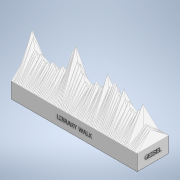
# Autodesk Inventor part: average_smplitude
Saved by Autodesk Inventor 2020 (Build 240168000, 168)
## iProperties
Created: 2019-09-30
Part Number: average_smplitude
Material: Generic
Document SubType Name: Modeling
Designer: Babynado
Density: 1 g/cm^3
Appearance: Default
Author: Babynado
Autodesk Inventor part; units mm, degrees
(part 1 of 3)
ref_plane "YZ Plane" through (0, 0, 0) normal (1, 0, 0) x (0, 1, 0)
ref_plane "XZ Plane" through (0, 0, 0) normal (0, 1, 0) x (-1, 0, 0)
ref_plane "XY Plane" through (0, 0, 0) normal (0, 0, 1) x (1, 0, 0)
sketch "Sketch1" plane through (0, 0, 0) normal (0, 1, 0) x (-1, 0, 0)
  line L0 (0, 0) -> (0, 50.8) projected
  line L1 (0, 50.8) -> (-203.2, 50.8) projected
  line L2 (-203.2, 50.8) -> (-203.2, 0) projected
  line L3 (-203.2, 0) -> (0, 0) projected
extrude "Extrusion1" add sketch "Sketch1" against normal blind 25.4
sketch "Sketch2" plane through (0, -25.4, 0) normal (0, -1, 0) x (1, 0, 0)
  line L0 (203.2, 0) -> (203.2, 50.8) projected
  line L1 (203.2, 50.8) -> (0, 50.8) projected
  line L2 (0, 50.8) -> (0, 0) projected
  line L3 (0, 0) -> (203.2, 0) projected
  line L4 (50.8, 29.464) -> (152.4, 29.464) construction
  line L5 (152.4, 29.464) -> (152.4, 21.336) construction
  line L6 (152.4, 21.336) -> (50.8, 21.336) construction
  line L7 (50.8, 21.336) -> (50.8, 29.464) construction
  spline S0 degree 2 poles (83.5812, 38.9215) (83.5812, 38.1212) (82.6031, 37.2517) (81.7781, 37.2517) knots 0 0 0 1 2 2 2
  spline S1 degree 2 poles (81.7781, 37.2517) (81.5805, 37.2517) (80.9235, 37.3209) (80.7012, 37.3703) knots 0 0 0 1 2 2 2
  line L8 (80.7012, 37.3703) -> (80.7012, 38.1508)
  line L9 (80.7012, 38.1508) -> (80.7457, 38.1508)
  spline S2 degree 2 poles (80.7457, 38.1508) (80.9136, 38.0915) (81.4126, 37.9532) (81.6694, 37.9532) knots 0 0 0 1 2 2 2
  spline S3 degree 2 poles (81.6694, 37.9532) (82.0449, 37.9532) (82.4944, 38.1261) (82.5982, 38.2842) knots 0 0 0 1 2 2 2
  spline S4 degree 2 poles (82.5982, 38.2842) (82.7118, 38.4472) (82.7711, 38.9215) (82.7711, 39.2327) knots 0 0 0 1 2 2 2
  line L10 (82.7711, 39.2327) -> (82.7711, 42.7846)
  line L11 (82.7711, 42.7846) -> (81.4817, 42.7846)
  line L12 (81.4817, 42.7846) -> (81.4817, 43.4317)
  line L13 (81.4817, 43.4317) -> (83.5812, 43.4317)
  line L14 (83.5812, 43.4317) -> (83.5812, 38.9215)
  line L15 (88.2743, 37.3357) -> (87.5036, 37.3357)
  line L16 (87.5036, 37.3357) -> (87.5036, 37.8396)
  spline S5 degree 2 poles (87.5036, 37.8396) (87.1479, 37.5284) (86.5107, 37.2073) (86.1155, 37.2073) knots 0 0 0 1 2 2 2
  spline S6 degree 2 poles (86.1155, 37.2073) (85.8191, 37.2073) (85.2905, 37.4049) (85.0978, 37.6173) knots 0 0 0 1 2 2 2
  spline S7 degree 2 poles (85.0978, 37.6173) (84.9002, 37.8297) (84.6829, 38.4769) (84.6829, 38.9412) knots 0 0 0 1 2 2 2
  line L17 (84.6829, 38.9412) -> (84.6829, 41.9102)
  line L18 (84.6829, 41.9102) -> (85.4535, 41.9102)
  line L19 (85.4535, 41.9102) -> (85.4535, 39.3019)
  spline S8 degree 2 poles (85.4535, 39.3019) (85.4535, 38.9363) (85.5078, 38.4571) (85.6017, 38.2793) knots 0 0 0 1 2 2 2
  spline S9 degree 2 poles (85.6017, 38.2793) (85.6956, 38.1014) (86.0167, 37.9384) (86.318, 37.9384) knots 0 0 0 1 2 2 2
  spline S10 degree 2 poles (86.318, 37.9384) (86.5996, 37.9384) (87.2369, 38.2595) (87.5036, 38.4917) knots 0 0 0 1 2 2 2
  line L20 (87.5036, 38.4917) -> (87.5036, 41.9102)
  line L21 (87.5036, 41.9102) -> (88.2743, 41.9102)
  line L22 (88.2743, 41.9102) -> (88.2743, 37.3357)
  spline S11 degree 2 poles (90.6257, 37.227) (90.1663, 37.227) (89.3709, 37.474) (89.1091, 37.6124) knots 0 0 0 1 2 2 2
  line L23 (89.1091, 37.6124) -> (89.1091, 38.4769)
  line L24 (89.1091, 38.4769) -> (89.1486, 38.4769)
  spline S12 degree 2 poles (89.1486, 38.4769) (89.2474, 38.3978) (89.5142, 38.2101) (89.7365, 38.1064) knots 0 0 0 1 2 2 2
  spline S13 degree 2 poles (89.7365, 38.1064) (89.9292, 38.0125) (90.4034, 37.8742) (90.6554, 37.8742) knots 0 0 0 1 2 2 2
  spline S14 degree 2 poles (90.6554, 37.8742) (90.8381, 37.8742) (91.258, 37.9582) (91.3568, 38.0273) knots 0 0 0 1 2 2 2
  spline S15 degree 2 poles (91.3568, 38.0273) (91.5001, 38.1212) (91.6285, 38.3336) (91.6285, 38.551) knots 0 0 0 1 2 2 2
  spline S16 degree 2 poles (91.6285, 38.551) (91.6285, 38.8227) (91.3321, 39.1043) (90.9518, 39.1981) knots 0 0 0 1 2 2 2
  spline S17 degree 2 poles (90.9518, 39.1981) (90.8036, 39.2327) (90.3293, 39.3315) (90.1268, 39.3858) knots 0 0 0 1 2 2 2
  spline S18 degree 2 poles (90.1268, 39.3858) (89.6031, 39.539) (89.1289, 40.1713) (89.1289, 40.6208) knots 0 0 0 1 2 2 2
  spline S19 degree 2 poles (89.1289, 40.6208) (89.1289, 41.2433) (90.0626, 42.0189) (90.8332, 42.0189) knots 0 0 0 1 2 2 2
  spline S20 degree 2 poles (90.8332, 42.0189) (91.2136, 42.0189) (91.9842, 41.8312) (92.246, 41.6879) knots 0 0 0 1 2 2 2
  line L25 (92.246, 41.6879) -> (92.246, 40.8629)
  line L26 (92.246, 40.8629) -> (92.2065, 40.8629)
  spline S21 degree 2 poles (92.2065, 40.8629) (91.9101, 41.1) (91.1889, 41.3717) (90.8184, 41.3717) knots 0 0 0 1 2 2 2
  spline S22 degree 2 poles (90.8184, 41.3717) (90.438, 41.3717) (89.9144, 41.0506) (89.9144, 40.7295) knots 0 0 0 1 2 2 2
  spline S23 degree 2 poles (89.9144, 40.7295) (89.9144, 40.4381) (90.2256, 40.1565) (90.5714, 40.0676) knots 0 0 0 1 2 2 2
  spline S24 degree 2 poles (90.5714, 40.0676) (90.7393, 40.0231) (91.1642, 39.9342) (91.3964, 39.8798) knots 0 0 0 1 2 2 2
  spline S25 degree 2 poles (91.3964, 39.8798) (91.9002, 39.7514) (92.414, 39.1635) (92.414, 38.6547) knots 0 0 0 1 2 2 2
  spline S26 degree 2 poles (92.414, 38.6547) (92.414, 38.3583) (92.1818, 37.8347) (91.9546, 37.642) knots 0 0 0 1 2 2 2
  spline S27 degree 2 poles (91.9546, 37.642) (91.7125, 37.4395) (91.095, 37.227) (90.6257, 37.227) knots 0 0 0 1 2 2 2
  spline S28 degree 2 poles (94.5135, 37.2468) (93.8861, 37.2468) (93.1797, 37.9631) (93.1797, 38.7387) knots 0 0 0 1 2 2 2
  line L27 (93.1797, 38.7387) -> (93.1797, 41.2729)
  line L28 (93.1797, 41.2729) -> (92.661, 41.2729)
  line L29 (92.661, 41.2729) -> (92.661, 41.9102)
  line L30 (92.661, 41.9102) -> (93.1797, 41.9102)
  line L31 (93.1797, 41.9102) -> (93.1797, 43.2242)
  line L32 (93.1797, 43.2242) -> (93.9504, 43.2242)
  line L33 (93.9504, 43.2242) -> (93.9504, 41.9102)
  line L34 (93.9504, 41.9102) -> (95.3681, 41.9102)
  line L35 (95.3681, 41.9102) -> (95.3681, 41.2729)
  line L36 (95.3681, 41.2729) -> (93.9504, 41.2729)
  line L37 (93.9504, 41.2729) -> (93.9504, 39.0944)
  spline S29 degree 2 poles (93.9504, 39.0944) (93.9504, 38.7486) (93.9751, 38.3682) (94.059, 38.2052) knots 0 0 0 1 2 2 2
  spline S30 degree 2 poles (94.059, 38.2052) (94.1282, 38.0619) (94.4394, 37.9186) (94.7062, 37.9186) knots 0 0 0 1 2 2 2
  spline S31 degree 2 poles (94.7062, 37.9186) (94.8939, 37.9186) (95.2446, 38.0323) (95.3237, 38.0668) knots 0 0 0 1 2 2 2
  line L38 (95.3237, 38.0668) -> (95.3681, 38.0668)
  line L39 (95.3681, 38.0668) -> (95.3681, 37.3752)
  spline S32 degree 2 poles (95.3681, 37.3752) (95.1508, 37.316) (94.7062, 37.2468) (94.5135, 37.2468) knots 0 0 0 1 2 2 2
  line L40 (96.7217, 37.3357) -> (95.9511, 37.3357)
  line L41 (95.9511, 37.3357) -> (95.9511, 41.9102)
  line L42 (95.9511, 41.9102) -> (96.7217, 41.9102)
  line L43 (96.7217, 41.9102) -> (96.7217, 37.3357)
  line L44 (96.7761, 42.671) -> (95.9017, 42.671)
  line L45 (95.9017, 42.671) -> (95.9017, 43.4712)
  line L46 (95.9017, 43.4712) -> (96.7761, 43.4712)
  line L47 (96.7761, 43.4712) -> (96.7761, 42.671)
  line L48 (101.4444, 37.3357) -> (100.6737, 37.3357)
  line L49 (100.6737, 37.3357) -> (100.6737, 39.9441)
  spline S33 degree 2 poles (100.6737, 39.9441) (100.6737, 40.2602) (100.6145, 40.8036) (100.5255, 40.9666) knots 0 0 0 1 2 2 2
  spline S34 degree 2 poles (100.5255, 40.9666) (100.4317, 41.1395) (100.0958, 41.3075) (99.8092, 41.3075) knots 0 0 0 1 2 2 2
  spline S35 degree 2 poles (99.8092, 41.3075) (99.5227, 41.3075) (98.9151, 41.0012) (98.6236, 40.7542) knots 0 0 0 1 2 2 2
  line L50 (98.6236, 40.7542) -> (98.6236, 37.3357)
  line L51 (98.6236, 37.3357) -> (97.853, 37.3357)
  line L52 (97.853, 37.3357) -> (97.853, 41.9102)
  line L53 (97.853, 41.9102) -> (98.6236, 41.9102)
  line L54 (98.6236, 41.9102) -> (98.6236, 41.4014)
  spline S36 degree 2 poles (98.6236, 41.4014) (98.9694, 41.7126) (99.6363, 42.0386) (100.0118, 42.0386) knots 0 0 0 1 2 2 2
  spline S37 degree 2 poles (100.0118, 42.0386) (100.6836, 42.0386) (101.4444, 41.1494) (101.4444, 40.3047) knots 0 0 0 1 2 2 2
  line L55 (101.4444, 40.3047) -> (101.4444, 37.3357)
  line L56 (104.5467, 37.3357) -> (106.6018, 43.4317)
  line L57 (106.6018, 43.4317) -> (107.5997, 43.4317)
  line L58 (107.5997, 43.4317) -> (109.6547, 37.3357)
  line L59 (109.6547, 37.3357) -> (108.8001, 37.3357)
  line L60 (108.8001, 37.3357) -> (108.2468, 39.04)
  line L61 (108.2468, 39.04) -> (105.9201, 39.04)
  line L62 (105.9201, 39.04) -> (105.3668, 37.3357)
  line L63 (105.3668, 37.3357) -> (104.5467, 37.3357)
  line L64 (108.0245, 39.7316) -> (107.081, 42.6018)
  line L65 (107.081, 42.6018) -> (106.1424, 39.7316)
  line L66 (106.1424, 39.7316) -> (108.0245, 39.7316)
  line L67 (110.9589, 37.3357) -> (110.1882, 37.3357)
  line L68 (110.1882, 37.3357) -> (110.1882, 43.7034)
  line L69 (110.1882, 43.7034) -> (110.9589, 43.7034)
  line L70 (110.9589, 43.7034) -> (110.9589, 37.3357)
  line L71 (112.8756, 37.3357) -> (112.105, 37.3357)
  line L72 (112.105, 37.3357) -> (112.105, 43.7034)
  line L73 (112.105, 43.7034) -> (112.8756, 43.7034)
  line L74 (112.8756, 43.7034) -> (112.8756, 37.3357)
  spline S38 degree 2 poles (115.9928, 37.232) (114.8961, 37.232) (113.6907, 38.4621) (113.6907, 39.5983) knots 0 0 0 1 2 2 2
  spline S39 degree 2 poles (113.6907, 39.5983) (113.6907, 40.7147) (114.8615, 42.0386) (115.8051, 42.0386) knots 0 0 0 1 2 2 2
  spline S40 degree 2 poles (115.8051, 42.0386) (116.2299, 42.0386) (116.8869, 41.7916) (117.129, 41.5298) knots 0 0 0 1 2 2 2
  spline S41 degree 2 poles (117.129, 41.5298) (117.376, 41.268) (117.6378, 40.5122) (117.6378, 39.9638) knots 0 0 0 1 2 2 2
  line L75 (117.6378, 39.9638) -> (117.6378, 39.5439)
  line L76 (117.6378, 39.5439) -> (114.4713, 39.5439)
  spline S42 degree 2 poles (114.4713, 39.5439) (114.4713, 38.7486) (115.2715, 37.9038) (115.9829, 37.9038) knots 0 0 0 1 2 2 2
  spline S43 degree 2 poles (115.9829, 37.9038) (116.2348, 37.9038) (116.7239, 38.0174) (116.9215, 38.1064) knots 0 0 0 1 2 2 2
  spline S44 degree 2 poles (116.9215, 38.1064) (117.129, 38.2052) (117.4155, 38.3781) (117.5094, 38.4571) knots 0 0 0 1 2 2 2
  line L77 (117.5094, 38.4571) -> (117.5538, 38.4571)
  line L78 (117.5538, 38.4571) -> (117.5538, 37.6173)
  spline S45 degree 2 poles (117.5538, 37.6173) (117.4205, 37.563) (117.0154, 37.4049) (116.8573, 37.3604) knots 0 0 0 1 2 2 2
  spline S46 degree 2 poles (116.8573, 37.3604) (116.635, 37.2962) (116.2694, 37.232) (115.9928, 37.232) knots 0 0 0 1 2 2 2
  spline S47 degree 2 poles (116.8869, 40.1318) (116.877, 40.443) (116.7486, 40.8975) (116.6251, 41.0506) knots 0 0 0 1 2 2 2
  spline S48 degree 2 poles (116.6251, 41.0506) (116.4917, 41.2235) (116.0718, 41.4063) (115.7606, 41.4063) knots 0 0 0 1 2 2 2
  spline S49 degree 2 poles (115.7606, 41.4063) (115.4543, 41.4063) (115.0245, 41.2235) (114.8467, 41.0457) knots 0 0 0 1 2 2 2
  spline S50 degree 2 poles (114.8467, 41.0457) (114.6738, 40.8629) (114.496, 40.4232) (114.4713, 40.1318) knots 0 0 0 1 2 2 2
  line L79 (114.4713, 40.1318) -> (116.8869, 40.1318)
  line L80 (122.0097, 37.3357) -> (121.2391, 37.3357)
  line L81 (121.2391, 37.3357) -> (121.2391, 39.9441)
  spline S51 degree 2 poles (121.2391, 39.9441) (121.2391, 40.2602) (121.1798, 40.8036) (121.0909, 40.9666) knots 0 0 0 1 2 2 2
  spline S52 degree 2 poles (121.0909, 40.9666) (120.997, 41.1395) (120.6611, 41.3075) (120.3746, 41.3075) knots 0 0 0 1 2 2 2
  spline S53 degree 2 poles (120.3746, 41.3075) (120.0881, 41.3075) (119.4804, 41.0012) (119.189, 40.7542) knots 0 0 0 1 2 2 2
  line L82 (119.189, 40.7542) -> (119.189, 37.3357)
  line L83 (119.189, 37.3357) -> (118.4183, 37.3357)
  line L84 (118.4183, 37.3357) -> (118.4183, 41.9102)
  line L85 (118.4183, 41.9102) -> (119.189, 41.9102)
  line L86 (119.189, 41.9102) -> (119.189, 41.4014)
  spline S54 degree 2 poles (119.189, 41.4014) (119.5348, 41.7126) (120.2017, 42.0386) (120.5771, 42.0386) knots 0 0 0 1 2 2 2
  spline S55 degree 2 poles (120.5771, 42.0386) (121.249, 42.0386) (122.0097, 41.1494) (122.0097, 40.3047) knots 0 0 0 1 2 2 2
  line L87 (122.0097, 40.3047) -> (122.0097, 37.3357)
  line L88 (80.7481, 27.2988) -> (82.8032, 33.3948)
  line L89 (82.8032, 33.3948) -> (83.8011, 33.3948)
  line L90 (83.8011, 33.3948) -> (85.8561, 27.2988)
  line L91 (85.8561, 27.2988) -> (85.0015, 27.2988)
  line L92 (85.0015, 27.2988) -> (84.4482, 29.0031)
  line L93 (84.4482, 29.0031) -> (82.1215, 29.0031)
  line L94 (82.1215, 29.0031) -> (81.5682, 27.2988)
  line L95 (81.5682, 27.2988) -> (80.7481, 27.2988)
  line L96 (84.2259, 29.6947) -> (83.2824, 32.5649)
  line L97 (83.2824, 32.5649) -> (82.3438, 29.6947)
  line L98 (82.3438, 29.6947) -> (84.2259, 29.6947)
  line L99 (89.7143, 27.2988) -> (86.7404, 27.2988)
  line L100 (86.7404, 27.2988) -> (86.7404, 27.9213)
  line L101 (86.7404, 27.9213) -> (87.8469, 27.9213)
  line L102 (87.8469, 27.9213) -> (87.8469, 32.0067)
  line L103 (87.8469, 32.0067) -> (86.7404, 32.0067)
  line L104 (86.7404, 32.0067) -> (86.7404, 32.5649)
  spline S56 degree 2 poles (86.7404, 32.5649) (87.3678, 32.5649) (87.9606, 32.9206) (88.0001, 33.4146) knots 0 0 0 1 2 2 2
  line L105 (88.0001, 33.4146) -> (88.6324, 33.4146)
  line L106 (88.6324, 33.4146) -> (88.6324, 27.9213)
  line L107 (88.6324, 27.9213) -> (89.7143, 27.9213)
  line L108 (89.7143, 27.9213) -> (89.7143, 27.2988)
  line L109 (94.7581, 29.3934) -> (94.0319, 29.3934)
  line L110 (94.0319, 29.3934) -> (94.0319, 27.2988)
  line L111 (94.0319, 27.2988) -> (93.2464, 27.2988)
  line L112 (93.2464, 27.2988) -> (93.2464, 29.3934)
  line L113 (93.2464, 29.3934) -> (90.5541, 29.3934)
  line L114 (90.5541, 29.3934) -> (90.5541, 30.253)
  line L115 (90.5541, 30.253) -> (93.281, 33.3948)
  line L116 (93.281, 33.3948) -> (94.0319, 33.3948)
  line L117 (94.0319, 33.3948) -> (94.0319, 30.0504)
  line L118 (94.0319, 30.0504) -> (94.7581, 30.0504)
  line L119 (94.7581, 30.0504) -> (94.7581, 29.3934)
  line L120 (93.2464, 30.0504) -> (93.2464, 32.4315)
  line L121 (93.2464, 32.4315) -> (91.1963, 30.0504)
  line L122 (91.1963, 30.0504) -> (93.2464, 30.0504)
  spline S57 degree 2 poles (99.1053, 29.2353) (99.1053, 28.7957) (98.8237, 28.0448) (98.5668, 27.7681) knots 0 0 0 1 2 2 2
  spline S58 degree 2 poles (98.5668, 27.7681) (98.3099, 27.4915) (97.5442, 27.1704) (97.07, 27.1704) knots 0 0 0 1 2 2 2
  spline S59 degree 2 poles (97.07, 27.1704) (96.6353, 27.1704) (95.7856, 27.363) (95.4744, 27.5162) knots 0 0 0 1 2 2 2
  line L123 (95.4744, 27.5162) -> (95.4744, 28.3807)
  line L124 (95.4744, 28.3807) -> (95.5336, 28.3807)
  spline S60 degree 2 poles (95.5336, 28.3807) (95.6275, 28.3115) (95.9782, 28.1337) (96.1907, 28.0546) knots 0 0 0 1 2 2 2
  spline S61 degree 2 poles (96.1907, 28.0546) (96.4327, 27.9707) (96.8329, 27.8768) (97.0848, 27.8768) knots 0 0 0 1 2 2 2
  spline S62 degree 2 poles (97.0848, 27.8768) (97.3318, 27.8768) (97.7962, 28.0546) (97.9641, 28.2473) knots 0 0 0 1 2 2 2
  spline S63 degree 2 poles (97.9641, 28.2473) (98.1173, 28.4301) (98.2754, 28.9142) (98.2754, 29.2403) knots 0 0 0 1 2 2 2
  spline S64 degree 2 poles (98.2754, 29.2403) (98.2754, 29.5663) (98.0975, 29.9813) (97.9296, 30.1196) knots 0 0 0 1 2 2 2
  spline S65 degree 2 poles (97.9296, 30.1196) (97.7567, 30.2727) (97.2429, 30.4012) (96.9317, 30.4012) knots 0 0 0 1 2 2 2
  spline S66 degree 2 poles (96.9317, 30.4012) (96.5957, 30.4012) (95.9288, 30.2974) (95.7263, 30.253) knots 0 0 0 1 2 2 2
  line L125 (95.7263, 30.253) -> (95.7263, 33.3948)
  line L126 (95.7263, 33.3948) -> (99.0707, 33.3948)
  line L127 (99.0707, 33.3948) -> (99.0707, 32.6785)
  line L128 (99.0707, 32.6785) -> (96.5118, 32.6785)
  line L129 (96.5118, 32.6785) -> (96.5118, 31.0532)
  spline S67 degree 2 poles (96.5118, 31.0532) (96.66, 31.073) (96.9465, 31.0878) (97.065, 31.0878) knots 0 0 0 1 2 2 2
  spline S68 degree 2 poles (97.065, 31.0878) (97.5344, 31.0878) (98.1815, 30.9347) (98.4779, 30.7074) knots 0 0 0 1 2 2 2
  spline S69 degree 2 poles (98.4779, 30.7074) (98.7792, 30.4802) (99.1053, 29.7886) (99.1053, 29.2353) knots 0 0 0 1 2 2 2
  spline S70 degree 2 poles (103.8378, 29.2748) (103.8378, 28.8055) (103.5266, 28.0102) (103.2648, 27.7434) knots 0 0 0 1 2 2 2
  spline S71 degree 2 poles (103.2648, 27.7434) (102.9931, 27.4618) (102.3114, 27.1704) (101.9013, 27.1704) knots 0 0 0 1 2 2 2
  spline S72 degree 2 poles (101.9013, 27.1704) (101.4913, 27.1704) (100.8145, 27.447) (100.5577, 27.7237) knots 0 0 0 1 2 2 2
  spline S73 degree 2 poles (100.5577, 27.7237) (100.2415, 28.0546) (99.8858, 29.1662) (99.8858, 29.9763) knots 0 0 0 1 2 2 2
  spline S74 degree 2 poles (99.8858, 29.9763) (99.8858, 30.7717) (100.2118, 32.0511) (100.5527, 32.5254) knots 0 0 0 1 2 2 2
  spline S75 degree 2 poles (100.5527, 32.5254) (100.8837, 32.9897) (101.931, 33.5084) (102.6176, 33.5084) knots 0 0 0 1 2 2 2
  spline S76 degree 2 poles (102.6176, 33.5084) (102.8202, 33.5084) (103.1759, 33.4689) (103.3093, 33.4245) knots 0 0 0 1 2 2 2
  line L130 (103.3093, 33.4245) -> (103.3093, 32.639)
  line L131 (103.3093, 32.639) -> (103.2747, 32.639)
  spline S77 degree 2 poles (103.2747, 32.639) (103.161, 32.6983) (102.7461, 32.802) (102.509, 32.802) knots 0 0 0 1 2 2 2
  spline S78 degree 2 poles (102.509, 32.802) (101.7482, 32.802) (100.8145, 31.7745) (100.7256, 30.7667) knots 0 0 0 1 2 2 2
  spline S79 degree 2 poles (100.7256, 30.7667) (101.0171, 30.9693) (101.6296, 31.1916) (101.9952, 31.1916) knots 0 0 0 1 2 2 2
  spline S80 degree 2 poles (101.9952, 31.1916) (102.3509, 31.1916) (102.8844, 31.0483) (103.1759, 30.8309) knots 0 0 0 1 2 2 2
  spline S81 degree 2 poles (103.1759, 30.8309) (103.5118, 30.579) (103.8378, 29.7985) (103.8378, 29.2748) knots 0 0 0 1 2 2 2
  spline S82 degree 2 poles (103.0079, 29.2403) (103.0079, 29.6157) (102.8103, 30.1245) (102.5929, 30.3024) knots 0 0 0 1 2 2 2
  spline S83 degree 2 poles (102.5929, 30.3024) (102.4299, 30.4308) (102.0248, 30.5148) (101.8124, 30.5148) knots 0 0 0 1 2 2 2
  spline S84 degree 2 poles (101.8124, 30.5148) (101.5259, 30.5148) (100.9874, 30.3419) (100.7256, 30.1789) knots 0 0 0 1 2 2 2
  spline S85 degree 2 poles (100.7256, 30.1789) (100.7207, 30.0899) (100.7108, 29.922) (100.7108, 29.7935) knots 0 0 0 1 2 2 2
  spline S86 degree 2 poles (100.7108, 29.7935) (100.7108, 29.1612) (100.9578, 28.3856) (101.1455, 28.1831) knots 0 0 0 1 2 2 2
  spline S87 degree 2 poles (101.1455, 28.1831) (101.3184, 27.9904) (101.6939, 27.8373) (101.9063, 27.8373) knots 0 0 0 1 2 2 2
  spline S88 degree 2 poles (101.9063, 27.8373) (102.4003, 27.8373) (103.0079, 28.5388) (103.0079, 29.2403) knots 0 0 0 1 2 2 2
  spline S89 degree 2 poles (108.4123, 29.2748) (108.4123, 28.8055) (108.1011, 28.0102) (107.8393, 27.7434) knots 0 0 0 1 2 2 2
  spline S90 degree 2 poles (107.8393, 27.7434) (107.5676, 27.4618) (106.8858, 27.1704) (106.4758, 27.1704) knots 0 0 0 1 2 2 2
  spline S91 degree 2 poles (106.4758, 27.1704) (106.0658, 27.1704) (105.389, 27.447) (105.1321, 27.7237) knots 0 0 0 1 2 2 2
  spline S92 degree 2 poles (105.1321, 27.7237) (104.816, 28.0546) (104.4603, 29.1662) (104.4603, 29.9763) knots 0 0 0 1 2 2 2
  spline S93 degree 2 poles (104.4603, 29.9763) (104.4603, 30.7717) (104.7863, 32.0511) (105.1272, 32.5254) knots 0 0 0 1 2 2 2
  spline S94 degree 2 poles (105.1272, 32.5254) (105.4582, 32.9897) (106.5055, 33.5084) (107.1921, 33.5084) knots 0 0 0 1 2 2 2
  spline S95 degree 2 poles (107.1921, 33.5084) (107.3947, 33.5084) (107.7503, 33.4689) (107.8837, 33.4245) knots 0 0 0 1 2 2 2
  line L132 (107.8837, 33.4245) -> (107.8837, 32.639)
  line L133 (107.8837, 32.639) -> (107.8491, 32.639)
  spline S96 degree 2 poles (107.8491, 32.639) (107.7355, 32.6983) (107.3206, 32.802) (107.0834, 32.802) knots 0 0 0 1 2 2 2
  spline S97 degree 2 poles (107.0834, 32.802) (106.3227, 32.802) (105.389, 31.7745) (105.3001, 30.7667) knots 0 0 0 1 2 2 2
  spline S98 degree 2 poles (105.3001, 30.7667) (105.5915, 30.9693) (106.2041, 31.1916) (106.5697, 31.1916) knots 0 0 0 1 2 2 2
  spline S99 degree 2 poles (106.5697, 31.1916) (106.9254, 31.1916) (107.4589, 31.0483) (107.7503, 30.8309) knots 0 0 0 1 2 2 2
  spline S100 degree 2 poles (107.7503, 30.8309) (108.0863, 30.579) (108.4123, 29.7985) (108.4123, 29.2748) knots 0 0 0 1 2 2 2
  spline S101 degree 2 poles (107.5824, 29.2403) (107.5824, 29.6157) (107.3848, 30.1245) (107.1674, 30.3024) knots 0 0 0 1 2 2 2
  spline S102 degree 2 poles (107.1674, 30.3024) (107.0044, 30.4308) (106.5993, 30.5148) (106.3869, 30.5148) knots 0 0 0 1 2 2 2
  spline S103 degree 2 poles (106.3869, 30.5148) (106.1004, 30.5148) (105.5619, 30.3419) (105.3001, 30.1789) knots 0 0 0 1 2 2 2
  spline S104 degree 2 poles (105.3001, 30.1789) (105.2951, 30.0899) (105.2853, 29.922) (105.2853, 29.7935) knots 0 0 0 1 2 2 2
  spline S105 degree 2 poles (105.2853, 29.7935) (105.2853, 29.1612) (105.5323, 28.3856) (105.72, 28.1831) knots 0 0 0 1 2 2 2
  spline S106 degree 2 poles (105.72, 28.1831) (105.8929, 27.9904) (106.2683, 27.8373) (106.4808, 27.8373) knots 0 0 0 1 2 2 2
  spline S107 degree 2 poles (106.4808, 27.8373) (106.9748, 27.8373) (107.5824, 28.5388) (107.5824, 29.2403) knots 0 0 0 1 2 2 2
  spline S108 degree 2 poles (112.9275, 30.3468) (112.9275, 28.7067) (111.9741, 27.1704) (110.9811, 27.1704) knots 0 0 0 1 2 2 2
  spline S109 degree 2 poles (110.9811, 27.1704) (109.9734, 27.1704) (109.0298, 28.7364) (109.0298, 30.3419) knots 0 0 0 1 2 2 2
  spline S110 degree 2 poles (109.0298, 30.3419) (109.0298, 31.9919) (109.9832, 33.5183) (110.9811, 33.5183) knots 0 0 0 1 2 2 2
  spline S111 degree 2 poles (110.9811, 33.5183) (111.9839, 33.5183) (112.9275, 31.9375) (112.9275, 30.3468) knots 0 0 0 1 2 2 2
  spline S112 degree 2 poles (111.8802, 28.4894) (111.9988, 28.7907) (112.0976, 29.7194) (112.0976, 30.3468) knots 0 0 0 1 2 2 2
  spline S113 degree 2 poles (112.0976, 30.3468) (112.0976, 30.9742) (111.9988, 31.898) (111.8753, 32.2092) knots 0 0 0 1 2 2 2
  spline S114 degree 2 poles (111.8753, 32.2092) (111.7518, 32.5204) (111.322, 32.8415) (110.9811, 32.8415) knots 0 0 0 1 2 2 2
  spline S115 degree 2 poles (110.9811, 32.8415) (110.6403, 32.8415) (110.2006, 32.5204) (110.0722, 32.1993) knots 0 0 0 1 2 2 2
  spline S116 degree 2 poles (110.0722, 32.1993) (109.9487, 31.8881) (109.8597, 30.9396) (109.8597, 30.3419) knots 0 0 0 1 2 2 2
  spline S117 degree 2 poles (109.8597, 30.3419) (109.8597, 29.6997) (109.9388, 28.8401) (110.0672, 28.5042) knots 0 0 0 1 2 2 2
  spline S118 degree 2 poles (110.0672, 28.5042) (110.1858, 28.188) (110.6254, 27.8472) (110.9811, 27.8472) knots 0 0 0 1 2 2 2
  spline S119 degree 2 poles (110.9811, 27.8472) (111.317, 27.8472) (111.7567, 28.1683) (111.8802, 28.4894) knots 0 0 0 1 2 2 2
  line L134 (117.5365, 32.4809) -> (114.8986, 27.2988)
  line L135 (114.8986, 27.2988) -> (114.0291, 27.2988)
  line L136 (114.0291, 27.2988) -> (116.8153, 32.6785)
  line L137 (116.8153, 32.6785) -> (113.6685, 32.6785)
  line L138 (113.6685, 32.6785) -> (113.6685, 33.3948)
  line L139 (113.6685, 33.3948) -> (117.5365, 33.3948)
  line L140 (117.5365, 33.3948) -> (117.5365, 32.4809)
  line L141 (121.7356, 27.2988) -> (118.7617, 27.2988)
  line L142 (118.7617, 27.2988) -> (118.7617, 27.9213)
  line L143 (118.7617, 27.9213) -> (119.8682, 27.9213)
  line L144 (119.8682, 27.9213) -> (119.8682, 32.0067)
  line L145 (119.8682, 32.0067) -> (118.7617, 32.0067)
  line L146 (118.7617, 32.0067) -> (118.7617, 32.5649)
  spline S120 degree 2 poles (118.7617, 32.5649) (119.3891, 32.5649) (119.9819, 32.9206) (120.0214, 33.4146) knots 0 0 0 1 2 2 2
  line L147 (120.0214, 33.4146) -> (120.6537, 33.4146)
  line L148 (120.6537, 33.4146) -> (120.6537, 27.9213)
  line L149 (120.6537, 27.9213) -> (121.7356, 27.9213)
  line L150 (121.7356, 27.9213) -> (121.7356, 27.2988)
  spline S121 degree 2 poles (70.8483, 17.1335) (70.8483, 16.353) (70.0085, 15.5329) (69.2724, 15.5329) knots 0 0 0 1 2 2 2
  spline S122 degree 2 poles (69.2724, 15.5329) (69.144, 15.5329) (68.8278, 15.5576) (68.6747, 15.5823) knots 0 0 0 1 2 2 2
  line L151 (68.6747, 15.5823) -> (68.6747, 16.2739)
  line L152 (68.6747, 16.2739) -> (68.7191, 16.2739)
  spline S123 degree 2 poles (68.7191, 16.2739) (68.8081, 16.2542) (69.0254, 16.2146) (69.1242, 16.2146) knots 0 0 0 1 2 2 2
  spline S124 degree 2 poles (69.1242, 16.2146) (69.4305, 16.2146) (69.8307, 16.3678) (69.9245, 16.5308) knots 0 0 0 1 2 2 2
  spline S125 degree 2 poles (69.9245, 16.5308) (70.0184, 16.679) (70.0777, 17.1285) (70.0777, 17.4496) knots 0 0 0 1 2 2 2
  line L153 (70.0777, 17.4496) -> (70.0777, 21.1991)
  line L154 (70.0777, 21.1991) -> (69.2527, 21.1991)
  line L155 (69.2527, 21.1991) -> (69.2527, 21.8364)
  line L156 (69.2527, 21.8364) -> (70.8483, 21.8364)
  line L157 (70.8483, 21.8364) -> (70.8483, 17.1335)
  line L158 (70.8532, 22.5972) -> (69.9789, 22.5972)
  line L159 (69.9789, 22.5972) -> (69.9789, 23.3974)
  line L160 (69.9789, 23.3974) -> (70.8532, 23.3974)
  line L161 (70.8532, 23.3974) -> (70.8532, 22.5972)
  spline S126 degree 2 poles (75.7982, 19.6233) (75.7982, 18.5019) (74.7114, 17.1335) (73.8914, 17.1335) knots 0 0 0 1 2 2 2
  spline S127 degree 2 poles (73.8914, 17.1335) (73.5209, 17.1335) (72.9923, 17.3163) (72.7354, 17.4743) knots 0 0 0 1 2 2 2
  line L162 (72.7354, 17.4743) -> (72.686, 17.2619)
  line L163 (72.686, 17.2619) -> (71.9647, 17.2619)
  line L164 (71.9647, 17.2619) -> (71.9647, 23.6296)
  line L165 (71.9647, 23.6296) -> (72.7354, 23.6296)
  line L166 (72.7354, 23.6296) -> (72.7354, 21.3572)
  spline S128 degree 2 poles (72.7354, 21.3572) (73.0269, 21.619) (73.7036, 21.9648) (74.1334, 21.9648) knots 0 0 0 1 2 2 2
  spline S129 degree 2 poles (74.1334, 21.9648) (74.909, 21.9648) (75.7982, 20.7249) (75.7982, 19.6233) knots 0 0 0 1 2 2 2
  spline S130 degree 2 poles (75.0029, 19.564) (75.0029, 20.384) (74.5039, 21.2337) (73.9506, 21.2337) knots 0 0 0 1 2 2 2
  spline S131 degree 2 poles (73.9506, 21.2337) (73.6394, 21.2337) (72.9972, 20.9373) (72.7354, 20.7101) knots 0 0 0 1 2 2 2
  line L167 (72.7354, 20.7101) -> (72.7354, 18.0869)
  spline S132 degree 2 poles (72.7354, 18.0869) (73.0269, 17.9436) (73.4764, 17.8251) (73.7432, 17.8251) knots 0 0 0 1 2 2 2
  spline S133 degree 2 poles (73.7432, 17.8251) (74.331, 17.8251) (75.0029, 18.6599) (75.0029, 19.564) knots 0 0 0 1 2 2 2
  spline S134 degree 2 poles (79.1476, 17.746) (79.0537, 17.6769) (78.7375, 17.4299) (78.5893, 17.3558) knots 0 0 0 1 2 2 2
  spline S135 degree 2 poles (78.5893, 17.3558) (78.3868, 17.2471) (78.0064, 17.1335) (77.6606, 17.1335) knots 0 0 0 1 2 2 2
  spline S136 degree 2 poles (77.6606, 17.1335) (77.379, 17.1335) (76.8702, 17.3459) (76.6775, 17.5386) knots 0 0 0 1 2 2 2
  spline S137 degree 2 poles (76.6775, 17.5386) (76.4948, 17.7263) (76.2725, 18.2796) (76.2725, 18.5858) knots 0 0 0 1 2 2 2
  spline S138 degree 2 poles (76.2725, 18.5858) (76.2725, 19.0601) (76.6726, 19.7319) (77.1073, 19.9246) knots 0 0 0 1 2 2 2
  spline S139 degree 2 poles (77.1073, 19.9246) (77.4926, 20.1024) (78.5399, 20.2358) (79.1476, 20.2704) knots 0 0 0 1 2 2 2
  line L168 (79.1476, 20.2704) -> (79.1476, 20.4186)
  spline S140 degree 2 poles (79.1476, 20.4186) (79.1476, 20.6854) (78.9845, 21.0163) (78.8363, 21.1102) knots 0 0 0 1 2 2 2
  spline S141 degree 2 poles (78.8363, 21.1102) (78.6881, 21.2041) (78.2633, 21.2633) (78.036, 21.2633) knots 0 0 0 1 2 2 2
  spline S142 degree 2 poles (78.036, 21.2633) (77.7693, 21.2633) (77.048, 21.1053) (76.6874, 20.9521) knots 0 0 0 1 2 2 2
  line L169 (76.6874, 20.9521) -> (76.643, 20.9521)
  line L170 (76.643, 20.9521) -> (76.643, 21.7376)
  spline S143 degree 2 poles (76.643, 21.7376) (76.8554, 21.7969) (77.6507, 21.9451) (78.041, 21.9451) knots 0 0 0 1 2 2 2
  spline S144 degree 2 poles (78.041, 21.9451) (78.5152, 21.9451) (79.1624, 21.7969) (79.4193, 21.6042) knots 0 0 0 1 2 2 2
  spline S145 degree 2 poles (79.4193, 21.6042) (79.6712, 21.4165) (79.9182, 20.8187) (79.9182, 20.389) knots 0 0 0 1 2 2 2
  line L171 (79.9182, 20.389) -> (79.9182, 17.2619)
  line L172 (79.9182, 17.2619) -> (79.1476, 17.2619)
  line L173 (79.1476, 17.2619) -> (79.1476, 17.746)
  line L174 (79.1476, 18.3882) -> (79.1476, 19.6578)
  spline S146 degree 2 poles (79.1476, 19.6578) (78.8709, 19.6331) (78.036, 19.5492) (77.7742, 19.4701) knots 0 0 0 1 2 2 2
  spline S147 degree 2 poles (77.7742, 19.4701) (77.4679, 19.3763) (77.0678, 18.986) (77.0678, 18.6402) knots 0 0 0 1 2 2 2
  spline S148 degree 2 poles (77.0678, 18.6402) (77.0678, 18.245) (77.5124, 17.8448) (77.9372, 17.8448) knots 0 0 0 1 2 2 2
  spline S149 degree 2 poles (77.9372, 17.8448) (78.2979, 17.8448) (78.8907, 18.1561) (79.1476, 18.3882) knots 0 0 0 1 2 2 2
  line L175 (81.7855, 17.2619) -> (81.0149, 17.2619)
  line L176 (81.0149, 17.2619) -> (81.0149, 23.6296)
  line L177 (81.0149, 23.6296) -> (81.7855, 23.6296)
  line L178 (81.7855, 23.6296) -> (81.7855, 17.2619)
  line L179 (83.7023, 17.2619) -> (82.9316, 17.2619)
  line L180 (82.9316, 17.2619) -> (82.9316, 23.6296)
  line L181 (82.9316, 23.6296) -> (83.7023, 23.6296)
  line L182 (83.7023, 23.6296) -> (83.7023, 17.2619)
  spline S150 degree 2 poles (86.8194, 17.1582) (85.7227, 17.1582) (84.5174, 18.3882) (84.5174, 19.5245) knots 0 0 0 1 2 2 2
  spline S151 degree 2 poles (84.5174, 19.5245) (84.5174, 20.6409) (85.6882, 21.9648) (86.6317, 21.9648) knots 0 0 0 1 2 2 2
  spline S152 degree 2 poles (86.6317, 21.9648) (87.0565, 21.9648) (87.7136, 21.7178) (87.9556, 21.456) knots 0 0 0 1 2 2 2
  spline S153 degree 2 poles (87.9556, 21.456) (88.2026, 21.1942) (88.4645, 20.4384) (88.4645, 19.89) knots 0 0 0 1 2 2 2
  line L183 (88.4645, 19.89) -> (88.4645, 19.4701)
  line L184 (88.4645, 19.4701) -> (85.2979, 19.4701)
  spline S154 degree 2 poles (85.2979, 19.4701) (85.2979, 18.6748) (86.0982, 17.83) (86.8095, 17.83) knots 0 0 0 1 2 2 2
  spline S155 degree 2 poles (86.8095, 17.83) (87.0615, 17.83) (87.5505, 17.9436) (87.7481, 18.0326) knots 0 0 0 1 2 2 2
  spline S156 degree 2 poles (87.7481, 18.0326) (87.9556, 18.1314) (88.2422, 18.3043) (88.336, 18.3833) knots 0 0 0 1 2 2 2
  line L185 (88.336, 18.3833) -> (88.3805, 18.3833)
  line L186 (88.3805, 18.3833) -> (88.3805, 17.5435)
  spline S157 degree 2 poles (88.3805, 17.5435) (88.2471, 17.4892) (87.842, 17.3311) (87.6839, 17.2866) knots 0 0 0 1 2 2 2
  spline S158 degree 2 poles (87.6839, 17.2866) (87.4616, 17.2224) (87.0961, 17.1582) (86.8194, 17.1582) knots 0 0 0 1 2 2 2
  spline S159 degree 2 poles (87.7136, 20.058) (87.7037, 20.3692) (87.5752, 20.8237) (87.4517, 20.9768) knots 0 0 0 1 2 2 2
  spline S160 degree 2 poles (87.4517, 20.9768) (87.3184, 21.1497) (86.8985, 21.3325) (86.5872, 21.3325) knots 0 0 0 1 2 2 2
  spline S161 degree 2 poles (86.5872, 21.3325) (86.281, 21.3325) (85.8512, 21.1497) (85.6733, 20.9719) knots 0 0 0 1 2 2 2
  spline S162 degree 2 poles (85.6733, 20.9719) (85.5004, 20.7891) (85.3226, 20.3494) (85.2979, 20.058) knots 0 0 0 1 2 2 2
  line L187 (85.2979, 20.058) -> (87.7136, 20.058)
  line L188 (92.8364, 17.2619) -> (92.0657, 17.2619)
  line L189 (92.0657, 17.2619) -> (92.0657, 19.8703)
  spline S163 degree 2 poles (92.0657, 19.8703) (92.0657, 20.1864) (92.0065, 20.7298) (91.9175, 20.8928) knots 0 0 0 1 2 2 2
  spline S164 degree 2 poles (91.9175, 20.8928) (91.8237, 21.0657) (91.4878, 21.2337) (91.2012, 21.2337) knots 0 0 0 1 2 2 2
  spline S165 degree 2 poles (91.2012, 21.2337) (90.9147, 21.2337) (90.3071, 20.9274) (90.0156, 20.6804) knots 0 0 0 1 2 2 2
  line L190 (90.0156, 20.6804) -> (90.0156, 17.2619)
  line L191 (90.0156, 17.2619) -> (89.245, 17.2619)
  line L192 (89.245, 17.2619) -> (89.245, 21.8364)
  line L193 (89.245, 21.8364) -> (90.0156, 21.8364)
  line L194 (90.0156, 21.8364) -> (90.0156, 21.3276)
  spline S166 degree 2 poles (90.0156, 21.3276) (90.3614, 21.6388) (91.0283, 21.9648) (91.4038, 21.9648) knots 0 0 0 1 2 2 2
  spline S167 degree 2 poles (91.4038, 21.9648) (92.0756, 21.9648) (92.8364, 21.0756) (92.8364, 20.2309) knots 0 0 0 1 2 2 2
  line L195 (92.8364, 20.2309) -> (92.8364, 17.2619)
  spline S168 degree 2 poles (100.4786, 19.9789) (100.4786, 19.4108) (100.1674, 18.3487) (99.8759, 17.9091) knots 0 0 0 1 2 2 2
  line L196 (99.8759, 17.9091) -> (98.1568, 17.9091)
  line L197 (98.1568, 17.9091) -> (98.0531, 18.3833)
  spline S169 degree 2 poles (98.0531, 18.3833) (97.7764, 18.1511) (97.317, 17.8745) (96.9168, 17.8745) knots 0 0 0 1 2 2 2
  spline S170 degree 2 poles (96.9168, 17.8745) (96.2895, 17.8745) (95.4842, 18.8872) (95.4842, 19.8456) knots 0 0 0 1 2 2 2
  spline S171 degree 2 poles (95.4842, 19.8456) (95.4842, 20.8089) (96.4722, 21.8808) (97.1095, 21.8808) knots 0 0 0 1 2 2 2
  spline S172 degree 2 poles (97.1095, 21.8808) (97.4059, 21.8808) (97.8308, 21.7326) (98.0481, 21.6091) knots 0 0 0 1 2 2 2
  line L198 (98.0481, 21.6091) -> (98.0481, 21.8067)
  line L199 (98.0481, 21.8067) -> (98.6953, 21.8067)
  line L200 (98.6953, 21.8067) -> (98.6953, 18.3635)
  line L201 (98.6953, 18.3635) -> (99.624, 18.3635)
  spline S173 degree 2 poles (99.624, 18.3635) (99.7821, 18.655) (99.9154, 19.5788) (99.9154, 19.9542) knots 0 0 0 1 2 2 2
  spline S174 degree 2 poles (99.9154, 19.9542) (99.9154, 21.293) (98.552, 22.9232) (97.2725, 22.9232) knots 0 0 0 1 2 2 2
  spline S175 degree 2 poles (97.2725, 22.9232) (96.0622, 22.9232) (94.4864, 21.1596) (94.4864, 19.8999) knots 0 0 0 1 2 2 2
  spline S176 degree 2 poles (94.4864, 19.8999) (94.4864, 18.5513) (96.0178, 16.8766) (97.2528, 16.8766) knots 0 0 0 1 2 2 2
  spline S177 degree 2 poles (97.2528, 16.8766) (97.5838, 16.8766) (98.3198, 16.9655) (98.6459, 17.0643) knots 0 0 0 1 2 2 2
  line L202 (98.6459, 17.0643) -> (98.6459, 16.4863)
  spline S178 degree 2 poles (98.6459, 16.4863) (98.3001, 16.4024) (97.5936, 16.3381) (97.2478, 16.3381) knots 0 0 0 1 2 2 2
  spline S179 degree 2 poles (97.2478, 16.3381) (95.8004, 16.3381) (93.8985, 18.329) (93.8985, 19.9098) knots 0 0 0 1 2 2 2
  spline S180 degree 2 poles (93.8985, 19.9098) (93.8985, 21.4115) (95.8597, 23.4765) (97.2676, 23.4765) knots 0 0 0 1 2 2 2
  spline S181 degree 2 poles (97.2676, 23.4765) (98.7743, 23.4765) (100.4786, 21.535) (100.4786, 19.9789) knots 0 0 0 1 2 2 2
  line L203 (98.0382, 18.9316) -> (98.0382, 21.0509)
  spline S182 degree 2 poles (98.0382, 21.0509) (97.811, 21.1695) (97.4257, 21.2732) (97.2133, 21.2732) knots 0 0 0 1 2 2 2
  spline S183 degree 2 poles (97.2133, 21.2732) (96.7489, 21.2732) (96.1857, 20.5816) (96.1857, 19.8554) knots 0 0 0 1 2 2 2
  spline S184 degree 2 poles (96.1857, 19.8554) (96.1857, 19.2034) (96.6106, 18.5068) (97.0799, 18.5068) knots 0 0 0 1 2 2 2
  spline S185 degree 2 poles (97.0799, 18.5068) (97.3269, 18.5068) (97.8159, 18.7439) (98.0382, 18.9316) knots 0 0 0 1 2 2 2
  line L204 (105.0975, 17.2619) -> (104.3269, 17.2619)
  line L205 (104.3269, 17.2619) -> (104.3269, 17.7658)
  spline S186 degree 2 poles (104.3269, 17.7658) (103.9712, 17.4546) (103.334, 17.1335) (102.9387, 17.1335) knots 0 0 0 1 2 2 2
  spline S187 degree 2 poles (102.9387, 17.1335) (102.6423, 17.1335) (102.1138, 17.3311) (101.9211, 17.5435) knots 0 0 0 1 2 2 2
  spline S188 degree 2 poles (101.9211, 17.5435) (101.7235, 17.7559) (101.5061, 18.4031) (101.5061, 18.8674) knots 0 0 0 1 2 2 2
  line L206 (101.5061, 18.8674) -> (101.5061, 21.8364)
  line L207 (101.5061, 21.8364) -> (102.2768, 21.8364)
  line L208 (102.2768, 21.8364) -> (102.2768, 19.2281)
  spline S189 degree 2 poles (102.2768, 19.2281) (102.2768, 18.8625) (102.3311, 18.3833) (102.425, 18.2055) knots 0 0 0 1 2 2 2
  spline S190 degree 2 poles (102.425, 18.2055) (102.5188, 18.0276) (102.8399, 17.8646) (103.1413, 17.8646) knots 0 0 0 1 2 2 2
  spline S191 degree 2 poles (103.1413, 17.8646) (103.4229, 17.8646) (104.0601, 18.1857) (104.3269, 18.4179) knots 0 0 0 1 2 2 2
  line L209 (104.3269, 18.4179) -> (104.3269, 21.8364)
  line L210 (104.3269, 21.8364) -> (105.0975, 21.8364)
  line L211 (105.0975, 21.8364) -> (105.0975, 17.2619)
  spline S192 degree 2 poles (108.0319, 17.1582) (107.5577, 17.1582) (106.7722, 17.4496) (106.4906, 17.746) knots 0 0 0 1 2 2 2
  spline S193 degree 2 poles (106.4906, 17.746) (106.2091, 18.0375) (105.8978, 18.9366) (105.8978, 19.5393) knots 0 0 0 1 2 2 2
  spline S194 degree 2 poles (105.8978, 19.5393) (105.8978, 20.142) (106.2189, 21.0213) (106.4906, 21.3177) knots 0 0 0 1 2 2 2
  spline S195 degree 2 poles (106.4906, 21.3177) (106.7623, 21.619) (107.5676, 21.9401) (108.0319, 21.9401) knots 0 0 0 1 2 2 2
  spline S196 degree 2 poles (108.0319, 21.9401) (108.4074, 21.9401) (109.1088, 21.7277) (109.3806, 21.5894) knots 0 0 0 1 2 2 2
  line L212 (109.3806, 21.5894) -> (109.3806, 20.7249)
  line L213 (109.3806, 20.7249) -> (109.3361, 20.7249)
  spline S197 degree 2 poles (109.3361, 20.7249) (109.2521, 20.794) (108.9952, 20.9719) (108.8124, 21.0657) knots 0 0 0 1 2 2 2
  spline S198 degree 2 poles (108.8124, 21.0657) (108.6494, 21.1448) (108.2147, 21.2683) (108.0171, 21.2683) knots 0 0 0 1 2 2 2
  spline S199 degree 2 poles (108.0171, 21.2683) (107.4194, 21.2683) (106.6932, 20.3643) (106.6932, 19.5393) knots 0 0 0 1 2 2 2
  spline S200 degree 2 poles (106.6932, 19.5393) (106.6932, 18.734) (107.3947, 17.83) (108.0171, 17.83) knots 0 0 0 1 2 2 2
  spline S201 degree 2 poles (108.0171, 17.83) (108.3925, 17.83) (109.0743, 18.1412) (109.3361, 18.3833) knots 0 0 0 1 2 2 2
  line L214 (109.3361, 18.3833) -> (109.3806, 18.3833)
  line L215 (109.3806, 18.3833) -> (109.3806, 17.5188)
  spline S202 degree 2 poles (109.3806, 17.5188) (109.2669, 17.4645) (108.9211, 17.3113) (108.7828, 17.2767) knots 0 0 0 1 2 2 2
  spline S203 degree 2 poles (108.7828, 17.2767) (108.5852, 17.2175) (108.274, 17.1582) (108.0319, 17.1582) knots 0 0 0 1 2 2 2
  spline S204 degree 2 poles (111.317, 17.1532) (110.8576, 17.1532) (110.0623, 17.4002) (109.8005, 17.5386) knots 0 0 0 1 2 2 2
  line L216 (109.8005, 17.5386) -> (109.8005, 18.4031)
  line L217 (109.8005, 18.4031) -> (109.84, 18.4031)
  spline S205 degree 2 poles (109.84, 18.4031) (109.9388, 18.324) (110.2055, 18.1363) (110.4278, 18.0326) knots 0 0 0 1 2 2 2
  spline S206 degree 2 poles (110.4278, 18.0326) (110.6205, 17.9387) (111.0947, 17.8004) (111.3467, 17.8004) knots 0 0 0 1 2 2 2
  spline S207 degree 2 poles (111.3467, 17.8004) (111.5295, 17.8004) (111.9494, 17.8844) (112.0482, 17.9535) knots 0 0 0 1 2 2 2
  spline S208 degree 2 poles (112.0482, 17.9535) (112.1914, 18.0474) (112.3199, 18.2598) (112.3199, 18.4772) knots 0 0 0 1 2 2 2
  spline S209 degree 2 poles (112.3199, 18.4772) (112.3199, 18.7489) (112.0235, 19.0304) (111.6431, 19.1243) knots 0 0 0 1 2 2 2
  spline S210 degree 2 poles (111.6431, 19.1243) (111.4949, 19.1589) (111.0206, 19.2577) (110.8181, 19.312) knots 0 0 0 1 2 2 2
  spline S211 degree 2 poles (110.8181, 19.312) (110.2945, 19.4652) (109.8202, 20.0975) (109.8202, 20.547) knots 0 0 0 1 2 2 2
  spline S212 degree 2 poles (109.8202, 20.547) (109.8202, 21.1695) (110.7539, 21.9451) (111.5245, 21.9451) knots 0 0 0 1 2 2 2
  spline S213 degree 2 poles (111.5245, 21.9451) (111.9049, 21.9451) (112.6756, 21.7573) (112.9374, 21.6141) knots 0 0 0 1 2 2 2
  line L218 (112.9374, 21.6141) -> (112.9374, 20.7891)
  line L219 (112.9374, 20.7891) -> (112.8979, 20.7891)
  spline S214 degree 2 poles (112.8979, 20.7891) (112.6015, 21.0262) (111.8802, 21.2979) (111.5097, 21.2979) knots 0 0 0 1 2 2 2
  spline S215 degree 2 poles (111.5097, 21.2979) (111.1293, 21.2979) (110.6057, 20.9768) (110.6057, 20.6557) knots 0 0 0 1 2 2 2
  spline S216 degree 2 poles (110.6057, 20.6557) (110.6057, 20.3643) (110.9169, 20.0827) (111.2627, 19.9938) knots 0 0 0 1 2 2 2
  spline S217 degree 2 poles (111.2627, 19.9938) (111.4307, 19.9493) (111.8555, 19.8604) (112.0877, 19.806) knots 0 0 0 1 2 2 2
  spline S218 degree 2 poles (112.0877, 19.806) (112.5916, 19.6776) (113.1053, 19.0897) (113.1053, 18.5809) knots 0 0 0 1 2 2 2
  spline S219 degree 2 poles (113.1053, 18.5809) (113.1053, 18.2845) (112.8732, 17.7609) (112.6459, 17.5682) knots 0 0 0 1 2 2 2
  spline S220 degree 2 poles (112.6459, 17.5682) (112.4039, 17.3657) (111.7863, 17.1532) (111.317, 17.1532) knots 0 0 0 1 2 2 2
  line L220 (117.3389, 17.2619) -> (116.5683, 17.2619)
  line L221 (116.5683, 17.2619) -> (116.5683, 17.7263)
  spline S221 degree 2 poles (116.5683, 17.7263) (116.3905, 17.5781) (116.1286, 17.3805) (115.9508, 17.2965) knots 0 0 0 1 2 2 2
  spline S222 degree 2 poles (115.9508, 17.2965) (115.7878, 17.2175) (115.437, 17.1335) (115.2048, 17.1335) knots 0 0 0 1 2 2 2
  spline S223 degree 2 poles (115.2048, 17.1335) (114.8294, 17.1335) (114.1971, 17.4447) (113.9748, 17.746) knots 0 0 0 1 2 2 2
  spline S224 degree 2 poles (113.9748, 17.746) (113.7525, 18.0474) (113.5055, 18.9366) (113.5055, 19.5146) knots 0 0 0 1 2 2 2
  spline S225 degree 2 poles (113.5055, 19.5146) (113.5055, 20.1173) (113.8167, 20.9966) (114.0884, 21.3276) knots 0 0 0 1 2 2 2
  spline S226 degree 2 poles (114.0884, 21.3276) (114.3403, 21.624) (115.0468, 21.9648) (115.437, 21.9648) knots 0 0 0 1 2 2 2
  spline S227 degree 2 poles (115.437, 21.9648) (115.7779, 21.9648) (116.2867, 21.8117) (116.5683, 21.6536) knots 0 0 0 1 2 2 2
  line L222 (116.5683, 21.6536) -> (116.5683, 23.6296)
  line L223 (116.5683, 23.6296) -> (117.3389, 23.6296)
  line L224 (117.3389, 23.6296) -> (117.3389, 17.2619)
  line L225 (116.5683, 18.3734) -> (116.5683, 21.0163)
  spline S228 degree 2 poles (116.5683, 21.0163) (116.2818, 21.1547) (115.8273, 21.2584) (115.5655, 21.2584) knots 0 0 0 1 2 2 2
  spline S229 degree 2 poles (115.5655, 21.2584) (114.9727, 21.2584) (114.3008, 20.3692) (114.3008, 19.5294) knots 0 0 0 1 2 2 2
  spline S230 degree 2 poles (114.3008, 19.5294) (114.3008, 18.7192) (114.8146, 17.8646) (115.3827, 17.8646) knots 0 0 0 1 2 2 2
  spline S231 degree 2 poles (115.3827, 17.8646) (115.684, 17.8646) (116.2966, 18.1412) (116.5683, 18.3734) knots 0 0 0 1 2 2 2
  line L226 (119.6509, 17.2619) -> (118.6728, 17.2619)
  line L227 (118.6728, 17.2619) -> (118.6728, 18.4278)
  line L228 (118.6728, 18.4278) -> (119.6509, 18.4278)
  line L229 (119.6509, 18.4278) -> (119.6509, 17.2619)
  spline S232 degree 2 poles (122.9805, 17.1582) (121.8838, 17.1582) (120.6784, 18.3882) (120.6784, 19.5245) knots 0 0 0 1 2 2 2
  spline S233 degree 2 poles (120.6784, 19.5245) (120.6784, 20.6409) (121.8492, 21.9648) (122.7927, 21.9648) knots 0 0 0 1 2 2 2
  spline S234 degree 2 poles (122.7927, 21.9648) (123.2176, 21.9648) (123.8746, 21.7178) (124.1167, 21.456) knots 0 0 0 1 2 2 2
  spline S235 degree 2 poles (124.1167, 21.456) (124.3637, 21.1942) (124.6255, 20.4384) (124.6255, 19.89) knots 0 0 0 1 2 2 2
  line L230 (124.6255, 19.89) -> (124.6255, 19.4701)
  line L231 (124.6255, 19.4701) -> (121.4589, 19.4701)
  spline S236 degree 2 poles (121.4589, 19.4701) (121.4589, 18.6748) (122.2592, 17.83) (122.9706, 17.83) knots 0 0 0 1 2 2 2
  spline S237 degree 2 poles (122.9706, 17.83) (123.2225, 17.83) (123.7116, 17.9436) (123.9092, 18.0326) knots 0 0 0 1 2 2 2
  spline S238 degree 2 poles (123.9092, 18.0326) (124.1167, 18.1314) (124.4032, 18.3043) (124.4971, 18.3833) knots 0 0 0 1 2 2 2
  line L232 (124.4971, 18.3833) -> (124.5415, 18.3833)
  line L233 (124.5415, 18.3833) -> (124.5415, 17.5435)
  spline S239 degree 2 poles (124.5415, 17.5435) (124.4081, 17.4892) (124.003, 17.3311) (123.845, 17.2866) knots 0 0 0 1 2 2 2
  spline S240 degree 2 poles (123.845, 17.2866) (123.6227, 17.2224) (123.2571, 17.1582) (122.9805, 17.1582) knots 0 0 0 1 2 2 2
  spline S241 degree 2 poles (123.8746, 20.058) (123.8647, 20.3692) (123.7363, 20.8237) (123.6128, 20.9768) knots 0 0 0 1 2 2 2
  spline S242 degree 2 poles (123.6128, 20.9768) (123.4794, 21.1497) (123.0595, 21.3325) (122.7483, 21.3325) knots 0 0 0 1 2 2 2
  spline S243 degree 2 poles (122.7483, 21.3325) (122.442, 21.3325) (122.0122, 21.1497) (121.8344, 20.9719) knots 0 0 0 1 2 2 2
  spline S244 degree 2 poles (121.8344, 20.9719) (121.6615, 20.7891) (121.4836, 20.3494) (121.4589, 20.058) knots 0 0 0 1 2 2 2
  line L234 (121.4589, 20.058) -> (123.8746, 20.058)
  line L235 (128.9233, 17.2619) -> (128.1527, 17.2619)
  line L236 (128.1527, 17.2619) -> (128.1527, 17.7263)
  spline S245 degree 2 poles (128.1527, 17.7263) (127.9748, 17.5781) (127.713, 17.3805) (127.5352, 17.2965) knots 0 0 0 1 2 2 2
  spline S246 degree 2 poles (127.5352, 17.2965) (127.3721, 17.2175) (127.0214, 17.1335) (126.7892, 17.1335) knots 0 0 0 1 2 2 2
  spline S247 degree 2 poles (126.7892, 17.1335) (126.4138, 17.1335) (125.7815, 17.4447) (125.5592, 17.746) knots 0 0 0 1 2 2 2
  spline S248 degree 2 poles (125.5592, 17.746) (125.3369, 18.0474) (125.0899, 18.9366) (125.0899, 19.5146) knots 0 0 0 1 2 2 2
  spline S249 degree 2 poles (125.0899, 19.5146) (125.0899, 20.1173) (125.4011, 20.9966) (125.6728, 21.3276) knots 0 0 0 1 2 2 2
  spline S250 degree 2 poles (125.6728, 21.3276) (125.9247, 21.624) (126.6311, 21.9648) (127.0214, 21.9648) knots 0 0 0 1 2 2 2
  spline S251 degree 2 poles (127.0214, 21.9648) (127.3623, 21.9648) (127.8711, 21.8117) (128.1527, 21.6536) knots 0 0 0 1 2 2 2
  line L237 (128.1527, 21.6536) -> (128.1527, 23.6296)
  line L238 (128.1527, 23.6296) -> (128.9233, 23.6296)
  line L239 (128.9233, 23.6296) -> (128.9233, 17.2619)
  line L240 (128.1527, 18.3734) -> (128.1527, 21.0163)
  spline S252 degree 2 poles (128.1527, 21.0163) (127.8662, 21.1547) (127.4117, 21.2584) (127.1498, 21.2584) knots 0 0 0 1 2 2 2
  spline S253 degree 2 poles (127.1498, 21.2584) (126.557, 21.2584) (125.8852, 20.3692) (125.8852, 19.5294) knots 0 0 0 1 2 2 2
  spline S254 degree 2 poles (125.8852, 19.5294) (125.8852, 18.7192) (126.399, 17.8646) (126.9671, 17.8646) knots 0 0 0 1 2 2 2
  spline S255 degree 2 poles (126.9671, 17.8646) (127.2684, 17.8646) (127.881, 18.1412) (128.1527, 18.3734) knots 0 0 0 1 2 2 2
  line L241 (133.5966, 17.2619) -> (132.8259, 17.2619)
  line L242 (132.8259, 17.2619) -> (132.8259, 17.7658)
  spline S256 degree 2 poles (132.8259, 17.7658) (132.4703, 17.4546) (131.833, 17.1335) (131.4378, 17.1335) knots 0 0 0 1 2 2 2
  spline S257 degree 2 poles (131.4378, 17.1335) (131.1414, 17.1335) (130.6128, 17.3311) (130.4201, 17.5435) knots 0 0 0 1 2 2 2
  spline S258 degree 2 poles (130.4201, 17.5435) (130.2225, 17.7559) (130.0052, 18.4031) (130.0052, 18.8674) knots 0 0 0 1 2 2 2
  line L243 (130.0052, 18.8674) -> (130.0052, 21.8364)
  line L244 (130.0052, 21.8364) -> (130.7758, 21.8364)
  line L245 (130.7758, 21.8364) -> (130.7758, 19.2281)
  spline S259 degree 2 poles (130.7758, 19.2281) (130.7758, 18.8625) (130.8302, 18.3833) (130.924, 18.2055) knots 0 0 0 1 2 2 2
  spline S260 degree 2 poles (130.924, 18.2055) (131.0179, 18.0276) (131.339, 17.8646) (131.6403, 17.8646) knots 0 0 0 1 2 2 2
  spline S261 degree 2 poles (131.6403, 17.8646) (131.9219, 17.8646) (132.5592, 18.1857) (132.8259, 18.4179) knots 0 0 0 1 2 2 2
  line L246 (132.8259, 18.4179) -> (132.8259, 21.8364)
  line L247 (132.8259, 21.8364) -> (133.5966, 21.8364)
  line L248 (133.5966, 21.8364) -> (133.5966, 17.2619)
  line L249 (69.9097, 7.225) -> (69.0995, 7.225)
  line L250 (69.0995, 7.225) -> (69.0995, 12.4763)
  line L251 (69.0995, 12.4763) -> (67.5088, 8.9046)
  line L252 (67.5088, 8.9046) -> (67.0148, 8.9046)
  line L253 (67.0148, 8.9046) -> (65.439, 12.4763)
  line L254 (65.439, 12.4763) -> (65.439, 7.225)
  line L255 (65.439, 7.225) -> (64.6831, 7.225)
  line L256 (64.6831, 7.225) -> (64.6831, 13.321)
  line L257 (64.6831, 13.321) -> (65.7897, 13.321)
  line L258 (65.7897, 13.321) -> (67.3112, 9.9272)
  line L259 (67.3112, 9.9272) -> (68.7834, 13.321)
  line L260 (68.7834, 13.321) -> (69.9097, 13.321)
  line L261 (69.9097, 13.321) -> (69.9097, 7.225)
  spline S262 degree 2 poles (73.2739, 7.0966) (72.7354, 7.0966) (71.9351, 7.3782) (71.6535, 7.6597) knots 0 0 0 1 2 2 2
  spline S263 degree 2 poles (71.6535, 7.6597) (71.3324, 7.9759) (71.0706, 8.8651) (71.0706, 9.5172) knots 0 0 0 1 2 2 2
  line L262 (71.0706, 9.5172) -> (71.0706, 13.321)
  line L263 (71.0706, 13.321) -> (71.8808, 13.321)
  line L264 (71.8808, 13.321) -> (71.8808, 9.5172)
  spline S264 degree 2 poles (71.8808, 9.5172) (71.8808, 9.0923) (71.9894, 8.5193) (72.1426, 8.2871) knots 0 0 0 1 2 2 2
  spline S265 degree 2 poles (72.1426, 8.2871) (72.3056, 8.0401) (72.8688, 7.7882) (73.2739, 7.7882) knots 0 0 0 1 2 2 2
  spline S266 degree 2 poles (73.2739, 7.7882) (73.6542, 7.7882) (74.247, 8.0401) (74.4101, 8.2871) knots 0 0 0 1 2 2 2
  spline S267 degree 2 poles (74.4101, 8.2871) (74.5632, 8.5193) (74.6719, 9.0874) (74.6719, 9.4974) knots 0 0 0 1 2 2 2
  line L265 (74.6719, 9.4974) -> (74.6719, 13.321)
  line L266 (74.6719, 13.321) -> (75.482, 13.321)
  line L267 (75.482, 13.321) -> (75.482, 9.5172)
  spline S268 degree 2 poles (75.482, 9.5172) (75.482, 8.8799) (75.2252, 7.971) (74.8991, 7.6597) knots 0 0 0 1 2 2 2
  spline S269 degree 2 poles (74.8991, 7.6597) (74.6077, 7.3732) (73.837, 7.0966) (73.2739, 7.0966) knots 0 0 0 1 2 2 2
  spline S270 degree 2 poles (78.3423, 7.1163) (77.6804, 7.1163) (76.7516, 7.393) (76.3416, 7.5906) knots 0 0 0 1 2 2 2
  line L268 (76.3416, 7.5906) -> (76.3416, 8.6082)
  line L269 (76.3416, 8.6082) -> (76.4009, 8.6082)
  spline S271 degree 2 poles (76.4009, 8.6082) (76.801, 8.2328) (77.8137, 7.8178) (78.283, 7.8178) knots 0 0 0 1 2 2 2
  spline S272 degree 2 poles (78.283, 7.8178) (78.9549, 7.8178) (79.6416, 8.376) (79.6416, 8.8355) knots 0 0 0 1 2 2 2
  spline S273 degree 2 poles (79.6416, 8.8355) (79.6416, 9.201) (79.2809, 9.6555) (78.8907, 9.7691) knots 0 0 0 1 2 2 2
  spline S274 degree 2 poles (78.8907, 9.7691) (78.6091, 9.8482) (78.1398, 9.9569) (77.789, 10.0458) knots 0 0 0 1 2 2 2
  spline S275 degree 2 poles (77.789, 10.0458) (77.4729, 10.1298) (76.9739, 10.3817) (76.7813, 10.5842) knots 0 0 0 1 2 2 2